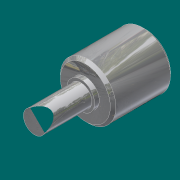
# Autodesk Inventor part: BRU-306_5
Saved by Autodesk Inventor 2016 (Build 200138000, 138)
## iProperties
Created: 2016-08-26
Part Number: BRU-306_5
Material: ステンレス鋼 AISI 304
Document SubType Name: Modeling
Designer: hiro
Density: 8 g/cm^3
Appearance: クローム - サテン
Mass: 1.51867 g
Surface Area: 2.43574 cm^2
Volume: 0.189834 cm^3
Author: hiro
Autodesk Inventor part; units mm, degrees
ref_plane "YZ Plane" through (0, 0, 0) normal (1, 0, 0) x (0, 1, 0)
ref_plane "XZ Plane" through (0, 0, 0) normal (0, 1, 0) x (-1, 0, 0)
ref_plane "XY Plane" through (0, 0, 0) normal (0, 0, 1) x (1, 0, 0)
sketch "スケッチ1" plane through (0, 0, 0) normal (0, 0, 1) x (1, 0, 0)
  line L0 (0, -4.25) -> (0.9, -4.25)
  line L1 (0.9, -4.25) -> (1.2, -3.95)
  line L2 (1.2, -3.95) -> (1.2, 1.25)
  line L3 (1.2, 1.25) -> (1.5, 1.25)
  line L4 (1.5, 1.25) -> (1.5, 1.75)
  line L5 (1.5, 1.75) -> (2.7, 1.75)
  line L6 (3, 7.95) -> (2.7, 8.25)
  line L7 (2.7, 8.25) -> (1.5, 8.25)
  line L8 (1.5, 8.25) -> (1.2, 7.95)
  line L9 (0, 7.4044) -> (0, -7.4044) construction
  line L10 (0, -4.25) -> (0, 4.25)
  line L11 (0, 4.25) -> (1.2, 4.25)
  line L12 (1.2, 4.25) -> (1.2, 7.95)
  line L13 (2.7, 1.75) -> (3, 2.05)
  line L14 (3, 2.05) -> (3, 7.95)
  point P0 (0, 0)
  point P1 (0, 0)
  dimension "d0" = 2.4
  dimension "d1" = 6
  dimension "d2" = 0.3
  dimension "d3" = 0.3
  dimension "d4" = 3
  dimension "d5" = 0.5
  dimension "d6" = 6.5
  dimension "d8" = 0.3
  dimension "d9" = 2.4
  dimension "d10" = 4
  dimension "d11" = 0.3
  dimension "d12" = 0.3
  dimension "d13" = 0.3
  dimension "d14" = 0.3
  dimension "d15" = 6
  constraints: 30 end point, 4 perpendicular, 4 vertical, 2 horizontal, 2 midpoint, 1 coincident, 1 collinear, 1 parallel
  measures "d0" diameter of L2 L9
  measures "d1" distance between parallel lines of L0 L5
  measures "d2" distance from line of L1.end L0
  measures "d3" horizontal distance of L1.end L0.end
  measures "d4" diameter of L4 L9
  measures "d5" distance of L3.end L4.end
  measures "d6" distance between parallel lines of L7 L5
  measures "d8" horizontal distance of L7.end L8.end
  measures "d9" diameter of L12 L9
  measures "d10" distance between parallel lines of L11 L7
  measures "d11" horizontal distance of L6.start L6.end
  measures "d12" horizontal distance of L6.start L6.end
  measures "d13" distance from line of L13.end L5
  measures "d14" horizontal distance of L5.end L13.end
  measures "d15" diameter of L14 L9
revolve "回転1" add sketch "スケッチ1" angle 360 about axis through (0, 7.4044, 0) along (0, -1, 0)
sketch "スケッチ2" plane through (0, -4.25, 0) normal (0, -1, 0) x (1, 0, 0)
  circle A0 centre (0, 0) radius 0.9 projected
  circle A1 centre (0, 0) radius 9.0242
  constraints: 1 centre point, 1 coincident
extrude "押し出し1" cut sketch "スケッチ2" against normal blind 0.5 contours A0 | A1
equation "\"d3\" = d2"
equation "\"d11\" = d8"
equation "\"d12\" = d8"
equation "\"d13\" = d12"
equation "\"d14\" = d13"
